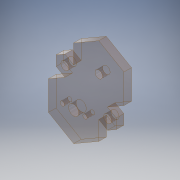
# Autodesk Inventor part: Dribbler Plate
Saved by Autodesk Inventor 2017 (Build 210142000, 142)
## iProperties
Created: 2017-04-14
Part Number: Dribbler Plate
Material: Polycarbonate, Smoke
Document SubType Name: Modeling
Designer: yella
Density: 1.2 g/cm^3
Appearance: Polycarbonate - Smoked
Author: yella
Autodesk Inventor part; units mm, degrees
ref_plane "YZ Plane" through (0, 0, 0) normal (1, 0, 0) x (0, 1, 0)
ref_plane "XZ Plane" through (0, 0, 0) normal (0, 1, 0) x (-1, 0, 0)
ref_plane "XY Plane" through (0, 0, 0) normal (0, 0, 1) x (1, 0, 0)
sketch "Sketch1" plane through (0, 0, 0) normal (0, 1, 0) x (-1, 0, 0)
  circle A0 centre (0, 0) radius 2.05
  line L0 (0, 0) -> (-4.5, 0)
  line L1 (0, 0) -> (4.5, 0)
  circle A1 centre (-4.5, 0) radius 0.85
  circle A2 centre (4.5, 0) radius 0.85
  line L2 (0, 0) -> (-5, 8.6603)
  line L3 (0, 0) -> (10, 0) construction
  line L4 (0, 11.547) -> (10, 5.7735)
  line L5 (10, 5.7735) -> (10, -5.7735)
  line L6 (10, -5.7735) -> (0, -11.547)
  line L7 (0, -11.547) -> (-10, -5.7735)
  line L8 (-10, -5.7735) -> (-10, 5.7735)
  line L9 (-10, 5.7735) -> (0, 11.547)
  line L10 (-5, 8.6603) -> (-10, 17.3205)
  line L11 (-10, 5.7735) -> (-20, 11.547)
  line L12 (-20, 11.547) -> (-20, 23.094)
  line L13 (-20, 23.094) -> (-10, 28.8675)
  line L14 (-10, 28.8675) -> (0, 23.094)
  line L15 (0, 23.094) -> (0, 11.547)
  line L16 (0, 11.547) -> (-10, 5.7735)
  circle A3 centre (-10, 17.3205) radius 1.5
  line L17 (-10, 5.7735) -> (-13.4641, 3.7735)
  line L18 (-13.4641, 3.7735) -> (0, 11.547)
  line L19 (0, 11.547) -> (3.4641, 13.547)
  line L20 (-10, 5.7735) -> (-10, 1.7735)
  line L21 (-10, 1.7735) -> (-13.4641, -0.2265)
  line L22 (-13.4641, -0.2265) -> (-16.9282, 1.7735)
  line L23 (-16.9282, 1.7735) -> (-16.9282, 5.7735)
  line L24 (-16.9282, 5.7735) -> (-13.4641, 7.7735)
  line L25 (-13.4641, 7.7735) -> (-10, 5.7735)
  line L26 (0, 11.547) -> (0, 15.547)
  line L27 (0, 15.547) -> (3.4641, 17.547)
  line L28 (3.4641, 17.547) -> (6.9282, 15.547)
  line L29 (6.9282, 15.547) -> (6.9282, 11.547)
  line L30 (6.9282, 11.547) -> (3.4641, 9.547)
  line L31 (3.4641, 9.547) -> (0, 11.547)
  circle A4 centre (-13.4641, 3.7735) radius 1.6
  circle A5 centre (3.4641, 13.547) radius 1.6
  dimension "d0" = 4.1
  dimension "d16" = 4.5
  dimension "d17" = 4.5
  dimension "d18" = 1.7
  dimension "d19" = 1.7
  dimension "d20" = 10
  dimension "d21" = 120
  dimension "d22" = 10
  dimension "d23" = 3
  dimension "d24" = 4
  dimension "d25" = 4
  dimension "d26" = 3.2
  dimension "d27" = 3.2
  constraints: 64 end point, 12 coincident, 6 centre point, 3 horizontal, 1 collinear, 1 equal length, 1 point on line, 52 other
  measures "d0" diameter of A0
  measures "d16" distance of L0.start L0.end
  measures "d17" distance of L0.start L1.end
  measures "d18" diameter of A1
  measures "d19" diameter of A2
  measures "d20" distance of L0.start L2.end
  measures "d21" angle of L3 L2
  measures "d22" distance of L2.end L10.end
  measures "d23" diameter of A3
  measures "d24" distance of L8.end L17.end
  measures "d25" distance of L15.end L19.end
  measures "d26" diameter of A4
  measures "d27" diameter of A5
extrude "Extrusion1" add sketch "Sketch1" along normal blind 3
body "Solid1"
